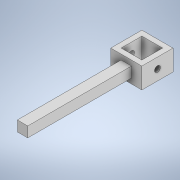
# Autodesk Inventor part: CAM02
Saved by Autodesk Inventor 2020.3 (Build 243373000, 373)
## iProperties
Created: 2021-05-24
Part Number: CAM02
Material: Generic
Document SubType Name: Modeling
Designer: patry
Density: 1 g/cm^3
Appearance: Default
Author: patry
Autodesk Inventor part; units mm, degrees
ref_plane "YZ Plane" through (0, 0, 0) normal (1, 0, 0) x (0, 1, 0)
ref_plane "XZ Plane" through (0, 0, 0) normal (0, 1, 0) x (-1, 0, 0)
ref_plane "XY Plane" through (0, 0, 0) normal (0, 0, 1) x (1, 0, 0)
sketch "Sketch1" plane through (0, 0, 0) normal (0, 1, 0) x (-1, 0, 0)
  line L0 (0, 0) -> (-15, 0)
  line L1 (-15, 0) -> (-15, 15)
  line L2 (-15, 15) -> (0, 15)
  line L3 (0, 15) -> (0, 0)
  line L4 (0, 0) -> (-2.5, 0)
  line L5 (-2.5, 0) -> (-2.5, 2.5)
  line L6 (-2.5, 2.5) -> (0, 2.5)
  line L7 (0, 2.5) -> (0, 0)
  line L8 (-2.5, 2.5) -> (-12.5, 2.5)
  line L9 (-12.5, 2.5) -> (-12.5, 12.5)
  line L10 (-12.5, 12.5) -> (-2.5, 12.5)
  line L11 (-2.5, 12.5) -> (-2.5, 2.5)
  dimension "d0" = 15
  dimension "d1" = 15
  dimension "d2" = 2.5
  dimension "d3" = 2.5
  dimension "d4" = 10
  dimension "d5" = 10
  constraints: 24 end point, 6 parallel, 3 horizontal, 3 perpendicular
  measures "d0" distance of L1.end L2.end
  measures "d1" distance of L0.end L1.end
  measures "d2" distance of L5.end L6.end
  measures "d3" distance of L4.end L5.end
  measures "d4" distance of L9.end L10.end
  measures "d5" distance of L8.end L9.end
extrude "Extrusion1" add sketch "Sketch1" along normal blind 10
sketch "Sketch2" plane through (15, 0, 15) normal (1, 0, 0) x (0, 0, -1)
  line L0 (15, 0) -> (15, 10) projected
  line L1 (0, 10) -> (15, 10)
  line L2 (15, 10) -> (15, 0)
  line L3 (15, 0) -> (0, 0)
  line L4 (0, 0) -> (0, 10)
  line L5 (0, 0) -> (0, 10) projected
  line L6 (0, 10) -> (7.5, 10)
  line L7 (7.5, 10) -> (7.5, 5)
  line L8 (7.5, 5) -> (0, 5)
  line L9 (0, 5) -> (0, 10)
  circle A0 centre (7.5, 5) radius 1.4
  dimension "d8" = 7.5
  dimension "d9" = 5
  dimension "d10" = 2.8
  constraints: 16 end point, 4 parallel, 2 horizontal, 2 perpendicular, 1 centre point, 1 coincident
  measures "d8" distance of L7.end L8.end
  measures "d9" distance of L6.end L7.end
  measures "d10" diameter of A0
extrude "Extrusion2" cut sketch "Sketch2" against normal through all contours A0 L8 L7 | L7 L8 A0
sketch "Sketch3" plane through (0, 0, 15) normal (0, 0, 1) x (1, 0, 0)
  line L0 (15, 10) -> (0, 10) projected
  line L1 (15, 0) -> (0, 0) projected
  line L2 (0, 10) -> (15, 10)
  line L3 (15, 10) -> (15, 0)
  line L4 (15, 0) -> (0, 0)
  line L5 (0, 0) -> (0, 10)
  line L6 (0, 10) -> (5, 10)
  line L7 (5, 10) -> (5, 7.5)
  line L8 (5, 7.5) -> (0, 7.5)
  line L9 (0, 7.5) -> (0, 10)
  line L10 (5, 7.5) -> (10, 7.5)
  line L11 (10, 7.5) -> (10, 2.5)
  line L12 (10, 2.5) -> (5, 2.5)
  line L13 (5, 2.5) -> (5, 7.5)
  dimension "d13" = 5
  dimension "d14" = 2.5
  dimension "d15" = 5
  dimension "d16" = 5
  constraints: 24 end point, 6 parallel, 3 horizontal, 3 perpendicular
  measures "d13" distance of L7.end L8.end
  measures "d14" distance of L6.end L7.end
  measures "d15" distance of L11.end L12.end
  measures "d16" distance of L10.end L11.end
extrude "Extrusion3" add sketch "Sketch3" along normal blind 50 contours L10 L11 L12 L13
body "Solid1"
